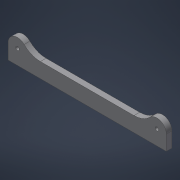
# Autodesk Inventor part: radiator_adapter_02
Saved by Autodesk Inventor 2022 (Build 260153000, 153)
## iProperties
Created: 2025-02-08
Part Number: radiator_adapter_02
Material: 一般
Document SubType Name: Modeling
Designer: gisen
Density: 1 g/cm^3
Appearance: 既定
Author: gisen
Autodesk Inventor part; units mm, degrees
ref_plane "YZ Plane" through (0, 0, 0) normal (1, 0, 0) x (0, 1, 0)
ref_plane "XZ Plane" through (0, 0, 0) normal (0, 1, 0) x (-1, 0, 0)
ref_plane "XY Plane" through (0, 0, 0) normal (0, 0, 1) x (1, 0, 0)
sketch "スケッチ2" plane through (0, 0, 0) normal (0, 0, 1) x (1, 0, 0)
  circle A0 centre (-61, -189) radius 2.1 construction
  circle A1 centre (61, -189) radius 2.1 construction
  arc A2 (66.8579, -183.1421) -> (55.1421, -183.1421) centre (61, -189) ccw
  arc A3 (41, -189) -> (55.1421, -183.1421) centre (41, -169) ccw
  line L0 (41, -189) -> (-41, -189)
  arc A4 (-55.1421, -183.1421) -> (-41, -189) centre (-41, -169) ccw
  arc A5 (-55.1421, -183.1421) -> (-66.8579, -183.1421) centre (-61, -189) ccw
  arc A6 (69.2843, -189) -> (66.8579, -183.1421) centre (61, -189) ccw
  arc A7 (-66.8579, -183.1421) -> (-69.2843, -189) centre (-61, -189) ccw
  line L1 (69.2843, -189) -> (69.2843, -202)
  line L2 (69.2843, -202) -> (-69.2843, -202)
  line L3 (-69.2843, -202) -> (-69.2843, -189)
  circle A8 centre (61, -189) radius 1.6
  circle A9 centre (-61, -189) radius 1.6
  point P0 (0, 0)
  point P1 (234, -202)
extrude "押し出し1" add sketch "スケッチ2" along normal blind 5
